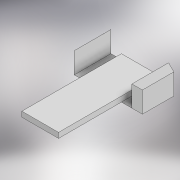
# Autodesk Inventor part: 부품2
Saved by Autodesk Inventor 2020 (Build 240168000, 168)
## iProperties
Created: 2022-04-05
Part Number: 부품2
Material: 일반
Document SubType Name: Modeling
Designer: Knowblesse
Density: 1 g/cm^3
Appearance: 기본값
Author: Knowblesse
## iProperties of the stored document _3D 인쇄.ipt
Created: 2022-04-05
Part Number: _3D 인쇄
Material: 일반
Document SubType Name: Modeling
Designer: Knowblesse
Density: 1 g/cm^3
Appearance: 기본값
Author: Knowblesse
Autodesk Inventor part; units mm, degrees
ref_plane "YZ Plane" through (0, 0, 0) normal (1, 0, 0) x (0, 1, 0)
ref_plane "XZ Plane" through (0, 0, 0) normal (0, 1, 0) x (-1, 0, 0)
ref_plane "XY Plane" through (0, 0, 0) normal (0, 0, 1) x (1, 0, 0)
sketch "스케치1" plane through (0, 0, 0) normal (0, 0, 1) x (1, 0, 0)
  line L0 (0, 5) -> (0, 0)
  line L1 (0, 0) -> (15.1186, 0)
  line L2 (0, 0) -> (13, 0)
  line L3 (13, 0) -> (13, 5)
  line L4 (13, 5) -> (12, 5)
  line L5 (12, 5) -> (12, 1)
  line L6 (12, 1) -> (1, 1)
  line L7 (1, 1) -> (1, 5)
  line L8 (1, 5) -> (0, 5)
  dimension "t" = 1
  dimension "d1" = 1
  dimension "d2" = 1
  dimension "d3" = 11
  dimension "d4" = 4
  constraints: 18 end point, 6 perpendicular, 2 vertical, 1 horizontal alignment, 1 point on line
  measures "t" distance of L7.end L0.start
  measures "d1" distance of L3.end L4.end
  measures "d2" distance between parallel lines of L6 L1
  measures "d3" distance of L5.end L6.end
  measures "d4" distance between parallel lines of L4 L6
extrude "돌출1" add sketch "스케치1" along normal blind 7
sketch "스케치2" plane through (1, 1, 0) normal (0, 1, 0) x (1, 0, 0)
  line L0 (11, 0) -> (0, 0) projected
  line L1 (0, 0) -> (0, -7) projected
  line L2 (11, 0) -> (11, -7) projected
  line L3 (9, 0) -> (2, 0)
  line L4 (2, 0) -> (2, -19)
  line L5 (2, -19) -> (9, -19)
  line L6 (9, -19) -> (9, 0)
  point P0 (-1, 0)
  point P1 (2, 0)
  dimension "d7" = 2
  dimension "d8" = 19
  dimension "d9" = 2
  constraints: 8 end point, 2 parallel, 1 horizontal, 1 perpendicular, 1 point on line
  measures "d7" distance between parallel lines of L2 L6
  measures "d8" distance of L3.end L4.end
  measures "d9" distance between parallel lines of L1 L4
extrude "돌출2" add sketch "스케치2" along normal blind 1
chamfer "모따기1" distance 1 angle 45 5 edges at (13, 5, 3.5) (6.5, 0, 7) (0, 5, 3.5) (13, 2.5, 7) (0, 2.5, 7)
equation "\"d1\" = t"
equation "\"d2\" = t"
